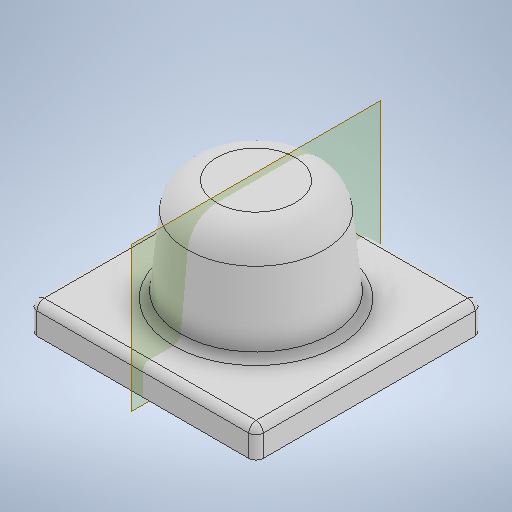
# Autodesk Inventor part: Part5
Saved by Autodesk Inventor 2025.1 (Build 291241000, 241)
## iProperties
Created: 2025-02-27
Part Number: Part5
Material: Generic
Document SubType Name: Modeling
Designer: santiago
Density: 1 g/cm^3
Appearance: Default
Author: santiago
Autodesk Inventor part; units mm, degrees
ref_plane "YZ Plane" through (0, 0, 0) normal (1, 0, 0) x (0, 1, 0)
ref_plane "XZ Plane" through (0, 0, 0) normal (0, 1, 0) x (-1, 0, 0)
ref_plane "XY Plane" through (0, 0, 0) normal (0, 0, 1) x (1, 0, 0)
sketch "Sketch1" plane through (0, 0, 0) normal (1, 0, 0) x (0, 1, 0)
  line L0 (9, 0) -> (9, 4.5)
  line L1 (9, 4.5) -> (2, 5.2)
  line L2 (2, 5.2) -> (2, 7.2)
  line L3 (2, 7.2) -> (0, 7.2)
  line L4 (0, 7.2) -> (0, 0)
  line L5 (9, 0) -> (0, 0)
  dimension "d0" = 4.5
  dimension "d1" = 9
  dimension "d2" = 2
  dimension "d3" = 2
  dimension "d5" = 7.2
  dimension "d6" = 5.2
  constraints: 12 end point, 2 perpendicular, 1 horizontal, 1 parallel, 1 vertical
  measures "d0" distance of L0.start L0.end
  measures "d1" distance between parallel lines of L4 L0
  measures "d2" distance between parallel lines of L4 L2
  measures "d3" distance of L1.end L2.end
  measures "d5" distance of L3.end L4.end
  measures "d6" distance from line of L5 L1.end
revolve "Revolution1" add sketch "Sketch1" angle 360 about axis through (0, 9, 0) along (0, -1, 0)
fillet "Fillet1" radius 2 1 edges at (0, 9, -4.5)
sketch "Sketch2" plane through (0, 0, 0) normal (0, -1, 0) x (1, 0, 0)
  line L0 (-7.75, -7.75) -> (7.75, -7.75)
  line L1 (7.75, -7.75) -> (7.75, 7.75)
  line L2 (7.75, 7.75) -> (-7.75, 7.75)
  line L3 (-7.75, 7.75) -> (-7.75, -7.75)
  line L4 (-7.75, -7.75) -> (7.75, 7.75) construction
  line L5 (7.75, -7.75) -> (-7.75, 7.75) construction
  point P0 (0, 0)
  dimension "d10" = 15.5
  dimension "d11" = 15.5
  constraints: 12 end point, 2 midpoint, 2 parallel, 1 horizontal, 1 perpendicular
  measures "d10" distance of L2.end L1.end
  measures "d11" distance of L1.end L0.end
extrude "Extrusion1" add sketch "Sketch2" against normal up to surface (2 mm away)
fillet "Fillet4" radius 0.5 9 edges at (7.75, 1, 7.75) (0, 2, 7.75) (-7.75, 2, 0) (0, 2, -7.75) (7.75, 2, 0) (0, 2, -5.2) (7.75, 1, -7.75) (-7.75, 1, -7.75) (-7.75, 1, 7.75)
ref_plane "Work Plane1" through (0, 0, -7.25) normal (-1, 0, 0) x (0, 0, 1)
body "Solid1"
